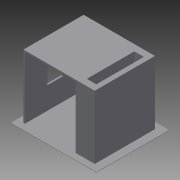
# Autodesk Inventor part: Bouchair_Solar_Chimney
Saved by Autodesk Inventor 2013 SP2 (Build 170200200, 200)
## iProperties
Created: 2015-11-25
Part Number: Bouchair_Solar_Chimney
Material: Generic
Document SubType Name: Modeling
Designer: mcgratta
Density: 1 g/cm^3
Author: mcgratta
Autodesk Inventor part; units mm, degrees
ref_plane "YZ Plane" through (0, 0, 0) normal (1, 0, 0) x (0, 1, 0)
ref_plane "XZ Plane" through (0, 0, 0) normal (0, 1, 0) x (-1, 0, 0)
ref_plane "XY Plane" through (0, 0, 0) normal (0, 0, 1) x (1, 0, 0)
sketch "Sketch2" plane through (0, 0, 0) normal (0, 1, 0) x (-1, 0, 0)
  line L0 (200, 200) -> (-2500, 200)
  line L1 (-2500, 200) -> (-2500, -2100)
  line L2 (-2500, -2100) -> (200, -2100)
  line L3 (200, -2100) -> (200, 200)
  point P0 (0, 0)
  dimension "d0" = 200
  dimension "d1" = 2300
  dimension "d2" = 2700
  dimension "d3" = 200
  constraints: 8 end point, 2 parallel, 1 horizontal, 1 perpendicular
  measures "d0" distance from line of point (0, 0) L0
  measures "d1" distance between parallel lines of L0 L2
  measures "d2" distance between parallel lines of L1 L3
  measures "d3" distance from line of point (0, 0) L3
extrude "Extrusion1" add sketch "Sketch2" against normal blind 10
sketch "Sketch3" plane through (0, 0, 0) normal (0, 1, 0) x (1, 0, 0)
  line L0 (1650, 0) -> (2250, 0)
  line L1 (2250, 0) -> (2250, 1900)
  line L2 (2250, 1900) -> (1650, 1900)
  line L3 (1650, 1900) -> (1650, 0)
  line L4 (0, 0) -> (50, 0)
  line L5 (50, 0) -> (50, 1900)
  line L6 (50, 1900) -> (0, 1900)
  line L7 (0, 1900) -> (0, 0)
  line L8 (50, 1900) -> (1650, 1900)
  line L9 (1650, 1900) -> (1650, 1850)
  line L10 (1650, 1850) -> (50, 1850)
  line L11 (50, 1850) -> (50, 1900)
  dimension "d6" = 1900
  dimension "d8" = 1900
  dimension "d9" = 1650
  dimension "d10" = 600
  dimension "d11" = 50
  dimension "d12" = 1900
  dimension "d13" = 50
  constraints: 24 end point, 6 parallel, 3 horizontal, 3 perpendicular, 1 point on line
  measures "d6" distance between parallel lines of L0 L2
  measures "d8" distance from line of L4.start L2
  measures "d9" distance from line of L3 L4.start
  measures "d10" distance between parallel lines of L1 L3
  measures "d11" distance between parallel lines of L5 L7
  measures "d12" distance from line of L4.start L6
  measures "d13" distance between parallel lines of L10 L8
extrude "Extrusion2" add sketch "Sketch3" along normal blind 2000
sketch "Sketch4" plane through (0, 2000, 0) normal (0, 1, 0) x (1, 0, 0)
  line L0 (1650, 1850) -> (1650, 0) projected
  line L1 (1650, 0) -> (2250, 0) projected
  line L2 (2250, 0) -> (2250, 1900) projected
  line L3 (2250, 1900) -> (0, 1900) projected
  line L4 (1800, 1700) -> (2100, 1700)
  line L5 (2100, 1700) -> (2100, 200)
  line L6 (2100, 200) -> (1800, 200)
  line L7 (1800, 200) -> (1800, 1700)
  dimension "d16" = 150
  dimension "d17" = 150
  dimension "d18" = 200
  dimension "d19" = 200
  constraints: 8 end point, 2 parallel, 1 horizontal, 1 perpendicular
  measures "d16" distance between parallel lines of L7 L0
  measures "d17" distance between parallel lines of L2 L5
  measures "d18" distance between parallel lines of L3 L4
  measures "d19" distance between parallel lines of L1 L6
extrude "Extrusion3" cut sketch "Sketch4" against normal blind 2000
sketch "Sketch5" plane through (1650, 0, -1850) normal (-1, 0, 0) x (0, 0, 1)
  line L0 (1850, 0) -> (0, 0) projected
  line L1 (1850, 0) -> (1850, 2000) projected
  line L2 (200, 0) -> (1600, 0)
  line L3 (1600, 0) -> (1600, 100)
  line L4 (1600, 100) -> (200, 100)
  line L5 (200, 100) -> (200, 0)
  dimension "d22" = 100
  dimension "d24" = 1400
  dimension "d25" = 250
  constraints: 8 end point, 2 parallel, 1 horizontal, 1 perpendicular, 1 point on line
  measures "d22" distance between parallel lines of L2 L4
  measures "d24" distance between parallel lines of L3 L5
  measures "d25" distance between parallel lines of L1 L3
extrude "Extrusion4" cut sketch "Sketch5" against normal blind 200
sketch "Sketch6" plane through (0, 0, -1900) normal (-1, 0, 0) x (0, 0, 1)
  line L0 (1900, 0) -> (0, 0) projected
  line L1 (0, 0) -> (0, 2000) projected
  line L2 (700, 1300) -> (1200, 1300)
  line L3 (1200, 1300) -> (1200, 700)
  line L4 (1200, 700) -> (700, 700)
  line L5 (700, 700) -> (700, 1300)
  dimension "d28" = 500
  dimension "d30" = 600
  dimension "d31" = 700
  dimension "d32" = 700
  constraints: 8 end point, 2 parallel, 1 horizontal, 1 perpendicular
  measures "d28" distance between parallel lines of L3 L5
  measures "d30" distance between parallel lines of L4 L2
  measures "d31" distance between parallel lines of L5 L1
  measures "d32" distance between parallel lines of L0 L4
extrude "Extrusion5" cut sketch "Sketch6" against normal blind 200
sketch "Sketch7" plane through (1650, 0, 0) normal (-1, 0, 0) x (0, 0, 1)
  line L0 (0, 0) -> (0, 2000) projected
  line L1 (-1850, 2000) -> (0, 2000)
  line L2 (0, 2000) -> (0, 1950)
  line L3 (0, 1950) -> (-1850, 1950)
  line L4 (-1850, 1950) -> (-1850, 2000)
  dimension "d35" = 50
  constraints: 8 end point, 2 parallel, 1 horizontal, 1 perpendicular, 1 point on line
  measures "d35" distance between parallel lines of L3 L1
extrude "Extrusion6" add sketch "Sketch7" along normal blind 1600
body "Solid1"
